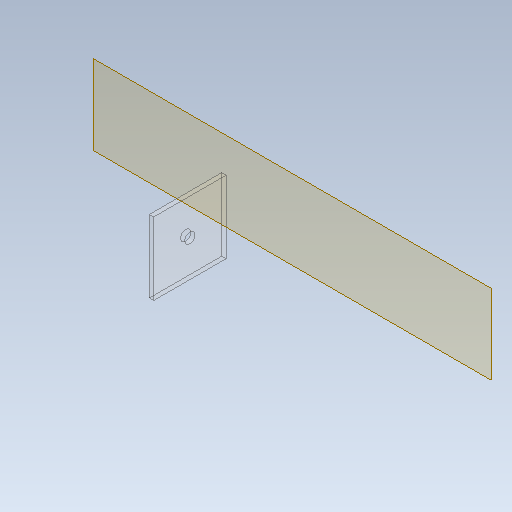
# Autodesk Inventor part: arm2
Saved by Autodesk Inventor 2021 (Build 250183000, 183)
## iProperties
Created: 2022-05-21
Part Number: arm2
Material: Polycarbonate, Clear
Document SubType Name: Modeling
Designer: techv
Mass: 8.86146 g
Surface Area: 55.89 cm^2
Volume: 7.38455 cm^3
Density: 1.2 g/cm^3
Appearance: Polycarbonate - Clear
Author: techv
Autodesk Inventor part; units mm, degrees
ref_plane "YZ Plane" through (0, 0, 0) normal (1, 0, 0) x (0, 1, 0)
ref_plane "XZ Plane" through (0, 0, 0) normal (0, 1, 0) x (-1, 0, 0)
ref_plane "XY Plane" through (0, 0, 0) normal (0, 0, 1) x (1, 0, 0)
ref_plane "Work Plane1" through (-10.1425, 21.3894, 8.8009) normal (0, 0, 1) x (1, 0, 0)
sketch "Sketch1" plane through (-10.1425, 21.3894, 8.8009) normal (0, 0, 1) x (1, 0, 0)
  line L0 (-48.6717, 3.6106) -> (201.3283, 3.6106) projected
  line L1 (-48.6717, -46.3894) -> (-48.6717, 3.6106) projected
  line L2 (201.3283, -46.3894) -> (-48.6717, -46.3894) projected
  line L3 (201.3283, 3.6106) -> (201.3283, -46.3894) projected
  circle A0 centre (172.519, -38.8894) radius 1.5 projected
  circle A1 centre (172.519, -3.8894) radius 1.5 projected
  circle A2 centre (195.2663, -38.8894) radius 1.5 projected
  circle A3 centre (195.2663, -3.8894) radius 1.5 projected
  line L4 (-48.6717, 3.6106) -> (-45.6717, 3.6106)
  line L5 (-45.6717, 3.6106) -> (-45.6717, -46.3894)
  line L6 (-45.6717, -46.3894) -> (-48.6717, -46.3894)
  line L7 (-48.6717, -46.3894) -> (-48.6717, 3.6106)
  point P0 (10.1425, -21.3894)
  point P1 (-45.6717, 3.6106)
  dimension "d0" = 3
  constraints: 8 end point, 2 parallel, 1 horizontal, 1 perpendicular, 1 point on line
  measures "d0" distance of L5.end L6.end
extrude "Extrusion1" add sketch "Sketch1" along normal blind 50 contours L0 L5 L2 L1
sketch "Sketch2" plane through (-58.8142, -25, 8.8009) normal (-1, 0, 0) x (0, 0, 1)
  line L0 (0, 50) -> (0, 0) projected
  line L1 (0, 0) -> (50, 0) projected
  line L2 (50, 50) -> (50, 0) projected
  line L3 (0, 50) -> (50, 50) projected
  circle A0 centre (25, 25) radius 3.5
  point P0 (-8.8009, 25)
  dimension "d3" = 7
  constraints: 1 centre point
  measures "d3" diameter of A0
extrude "Extrusion2" cut sketch "Sketch2" against normal through all contours A0
body "Solid1"
